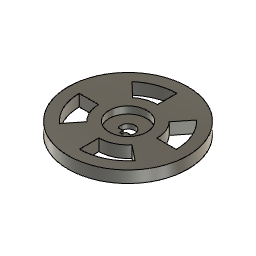
rotart+encoder+wheel (Autodesk Fusion 360 design; units mm, degrees)
Autodesk Fusion 360 part; units mm, degrees
sketch "Sketch1" plane through (0, 0, 0) normal (0, 0, 1) x (1, 0, 0)
  circle A0 centre (0, 0) radius 25.4
  line L0 (-0.4775, -1.5) -> (-2.5981, -1.5)
  line L1 (0.4974, -1.5) -> (2.5981, -1.5)
  line L2 (-0.4775, -1.5) -> (-0.4775, -2.9618)
  line L3 (0.4974, -1.5) -> (0.4974, -2.9585)
  arc A1 (-0.4775, -2.9618) -> (0.4974, -2.9585) centre (0, 0) ccw
  arc A2 (2.5981, -1.5) -> (-2.5981, -1.5) centre (0, 0) ccw
  dimension "d1" = 6
  dimension "d2" = 50.8
  constraint coincident A0.centre A1.centre
  constraint coincident L1.end A1
  constraint perpendicular L0 L2
  constraint perpendicular L1 L3
  constraint concentric A1 A2
  measures "d1" diameter of A1
  measures "d2" diameter of A0
extrude "Extrude1" add sketch "Sketch1" along normal blind 5
sketch "Sketch2" plane through (0, 0, 5) normal (0, 0, 1) x (-1, 0, 0)
  line L0 (-2.5981, 1.5) -> (-0.4974, 1.5)
  line L1 (-0.4974, 1.5) -> (-0.4974, 2.9585)
  arc A0 (0.4775, 2.9618) -> (-0.4974, 2.9585) centre (0, 0) ccw
  line L2 (0.4775, 2.9618) -> (0.4775, 1.5)
  line L3 (0.4775, 1.5) -> (2.5981, 1.5)
  arc A1 (-2.5981, 1.5) -> (2.5981, 1.5) centre (0, 0) ccw
  circle A2 centre (0, 0) radius 25.4
  circle A3 centre (0, 0) radius 8
  dimension "d6" = 16
  constraint concentric A0 A3
  measures "d6" diameter of A3
extrude "Extrude2" cut sketch "Sketch2" against normal blind 3 contours A3
sketch "Sketch3" plane through (0, 0, 5) normal (0, 0, 1) x (-1, 0, 0)
  circle A0 centre (0, 0) radius 8
  circle A1 centre (0, 0) radius 25.4
  circle A2 centre (0, 0) radius 12.3693
  circle A3 centre (0, 0) radius 20.6155
  line L0 (12.3686, 0.1302) -> (20.6151, 0.1302)
  line L1 (7.7191, -9.6651) -> (13.7003, -15.4046)
  line L2 (-0.1309, -12.3686) -> (-0.1309, -20.6151)
  line L3 (-12.3686, 0.1298) -> (-20.6151, 0.1298)
  line L4 (0, 12.3693) -> (0, 20.6155)
  line L5 (8.5619, 8.9272) -> (13.7135, 15.3929)
  line L6 (-9.5501, 7.861) -> (-16, 13)
  line L7 (-8.971, -8.5159) -> (-14.1393, -15.0026)
  constraint concentric A0 A2
  constraint concentric A0 A3
  constraint coincident A2 L0.start
  constraint coincident A3 L0.end
  constraint horizontal L0
  constraint coincident A2 L1.start
  constraint coincident A3 L1.end
  constraint coincident A2 L2.start
  constraint coincident A3 L2.end
  constraint vertical L2
  constraint coincident A2 L3.start
  constraint coincident A3 L3.end
  constraint perpendicular L2 L3
  constraint coincident A2 L4.start
  constraint coincident A3 L4.end
  constraint vertical L4
  constraint coincident A2 L5.start
  constraint coincident A3 L5.end
  constraint coincident A2 L6.start
  constraint coincident A3 L6.end
  constraint perpendicular L5 L6
  constraint coincident A2 L7.start
  constraint coincident A3 L7.end
  constraint perpendicular L6 L7
extrude "Extrude3" cut sketch "Sketch3" against normal blind 5 contours A2 A3 L0 L5 | A2 A3 L1 L2 | A2 A3 L4 L6 | A2 A3 L3 L7
